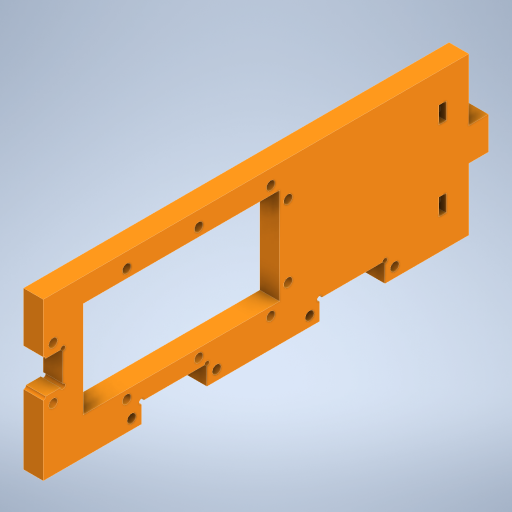
# Autodesk Inventor part: frame_upper2
Saved by Autodesk Inventor 2024 (Build 280153000, 153)
## iProperties
Created: 2024-09-07
Part Number: frame_upper2
Material: PMMA 플라스틱
Document SubType Name: Modeling
Designer: jmha0
Density: 1.188 g/cm^3
Appearance: 주황색
Mass: 30.1586 g
Surface Area: 129.801 cm^2
Volume: 25.386 cm^3
Author: jmha0
Autodesk Inventor part; units mm, degrees
ref_plane "YZ Plane" through (0, 0, 0) normal (1, 0, 0) x (0, 1, 0)
ref_plane "XZ Plane" through (0, 0, 0) normal (0, 1, 0) x (-1, 0, 0)
ref_plane "XY Plane" through (0, 0, 0) normal (0, 0, 1) x (1, 0, 0)
sketch "스케치1" plane through (0, 0, 0) normal (1, 0, 0) x (0, 1, 0)
  line L0 (5.1918, 130.7121) -> (5.1918, 0.7121)
  line L1 (5.1918, 0.7121) -> (11.1918, 0.7121)
  line L2 (11.1918, 130.7121) -> (11.1918, 0.7121)
  line L3 (5.1918, 130.7121) -> (11.1918, 130.7121)
  arc A0 (51.3918, 105.7888) -> (50.8725, 107.4757) centre (48.3918, 105.7888) ccw
  line L4 (50.8725, 107.4757) -> (46.887, 113.3367)
  line L5 (15.6965, 113.3367) -> (11.711, 107.4757)
  arc A1 (11.711, 107.4757) -> (11.1918, 105.7888) centre (14.1918, 105.7888) ccw
  line L6 (11.1918, 105.7888) -> (11.1918, 61.5355)
  arc A2 (11.1918, 61.5355) -> (11.711, 59.8486) centre (14.1918, 61.5355) ccw
  line L7 (11.711, 59.8486) -> (15.3989, 54.4252)
  arc A3 (15.3989, 54.4252) -> (17.8797, 53.1121) centre (17.8797, 56.1121) ccw
  line L8 (17.8797, 53.1121) -> (44.7039, 53.1121)
  arc A4 (44.7039, 53.1121) -> (47.1846, 54.4252) centre (44.7039, 56.1121) ccw
  line L9 (47.1846, 54.4252) -> (50.8725, 59.8486)
  arc A5 (50.8725, 59.8486) -> (51.3918, 61.5355) centre (48.3918, 61.5355) ccw
  line L10 (51.3918, 61.5355) -> (51.3918, 105.7888)
  circle A6 centre (48.5918, 105.2121) radius 1.45
  circle A7 centre (48.5918, 83.2121) radius 1.45
  circle A8 centre (48.5918, 61.2121) radius 1.45
  circle A9 centre (42.2918, 55.9121) radius 1.45
  circle A10 centre (20.2918, 55.9121) radius 1.45
  circle A11 centre (13.9918, 61.2121) radius 1.45
  circle A12 centre (13.9918, 83.2121) radius 1.45
  circle A13 centre (13.9918, 105.2121) radius 1.45
  line L11 (16.5918, 112.7121) -> (16.5918, 59.7121)
  arc A14 (16.5918, 59.7121) -> (17.7918, 58.5121) centre (17.7918, 59.7121) ccw
  line L12 (17.7918, 58.5121) -> (44.7918, 58.5121)
  arc A15 (44.7918, 58.5121) -> (45.9918, 59.7121) centre (44.7918, 59.7121) ccw
  line L13 (45.9918, 59.7121) -> (45.9918, 112.7121)
  line L14 (11.1918, 130.7121) -> (53.1918, 130.7121)
  line L15 (53.1918, 130.7121) -> (53.1918, 0.7121)
  line L16 (53.1918, 0.7121) -> (11.1918, 0.7121)
  line L17 (11.1918, 0.7121) -> (11.1918, 130.7121)
  line L18 (45.9918, 58.5121) -> (16.5918, 58.5121)
  line L19 (16.5918, 58.5121) -> (16.5918, 118.5121)
  line L20 (16.5918, 118.5121) -> (45.9918, 118.5121)
  line L21 (45.9918, 118.5121) -> (45.9918, 58.5121)
  circle A16 centre (48.5918, 105.2121) radius 1.35
  circle A17 centre (48.5918, 83.2121) radius 1.35
  circle A18 centre (48.5918, 61.2121) radius 1.35
  circle A19 centre (42.2918, 55.9121) radius 1.35
  circle A20 centre (20.2918, 55.9121) radius 1.35
  circle A21 centre (13.9918, 61.2121) radius 1.35
  circle A22 centre (13.9918, 83.2121) radius 1.35
  circle A23 centre (13.9918, 105.2121) radius 1.35
  point P0 (31.2918, 101.2121)
  point P1 (32.1918, 130.7121)
  point P2 (45.9918, 59.7121)
  point P3 (17.7918, 58.5121)
  dimension "d9" = 42
  dimension "d10" = 130
  dimension "d11" = 60
  dimension "d12" = 12.2
  dimension "d62" = 0.1
  dimension "d63" = 0.1
  dimension "d64" = 0.1
  dimension "d65" = 0.1
  dimension "d66" = 0.1
  dimension "d67" = 0.1
  dimension "d68" = 0.1
  dimension "d69" = 0.1
  constraints: 44 end point, 24 centre point, 16 point on circle, 4 parallel, 2 perpendicular, 2 point on line, 1 horizontal, 1 midpoint
  measures "d9" distance of L15.end L16.end
  measures "d10" distance of L14.end L15.end
  measures "d11" distance of L18.end L19.end
  measures "d12" distance from line of point (32.192, 130.712) L20
  measures "d62" radial gap between concentric circles of A6 A16
  measures "d63" radial gap between concentric circles of A7 A17
  measures "d64" radial gap between concentric circles of A8 A18
  measures "d65" radial gap between concentric circles of A9 A19
  measures "d66" radial gap between concentric circles of A10 A20
  measures "d67" radial gap between concentric circles of A11 A21
  measures "d68" radial gap between concentric circles of A12 A22
  measures "d69" radial gap between concentric circles of A13 A23
extrude "돌출1" add sketch "스케치1" along normal blind 6 contours L3 L2 L1 L0 | L14 L15 L16 L2 | A6 | A7 | A8 | A9 | A10 | A11 | A12 | A13
sketch "스케치3" plane through (6, 0, 0) normal (1, 0, 0) x (0, 0, -1)
  line L0 (-58.5121, 16.5918) -> (-118.5121, 16.5918) projected
  line L1 (-58.5121, 16.5918) -> (-46.3121, 16.5918)
  line L2 (-130.7121, 5.1918) -> (-0.7121, 5.1918) projected
  line L3 (-46.3121, 5.1918) -> (-26.3121, 5.1918)
  line L4 (-26.3121, 5.1918) -> (-26.3121, 11.1918)
  line L5 (-26.3121, 11.1918) -> (-46.3121, 11.1918)
  line L6 (-46.3121, 11.1918) -> (-46.3121, 5.1918)
  line L7 (-130.7121, 53.1918) -> (-130.7121, 5.1918) projected
  line L8 (-130.7121, 53.1918) -> (-130.7121, 32.1918)
  line L9 (-130.7121, 32.1918) -> (-124.7121, 32.1918)
  line L10 (-124.7121, 32.1918) -> (-124.7121, 42.1918)
  line L11 (-124.7121, 42.1918) -> (-130.7121, 42.1918)
  line L12 (-130.7121, 42.1918) -> (-130.7121, 32.1918)
  line L13 (-124.7121, 32.1918) -> (-130.7121, 32.1918)
  line L14 (-130.7121, 32.1918) -> (-130.7121, 22.1918)
  line L15 (-130.7121, 22.1918) -> (-124.7121, 22.1918)
  line L16 (-124.7121, 22.1918) -> (-124.7121, 32.1918)
  point P0 (0, 0)
  point P1 (-46.3121, 8.1918)
  dimension "d20" = 12.2
  dimension "d21" = 20
  dimension "d22" = 6
  dimension "d25" = 84.4
  dimension "d26" = 48
  dimension "d27" = 21
  dimension "d28" = 6
  dimension "d29" = 10
  dimension "d30" = 10
  constraints: 28 end point, 6 parallel, 4 horizontal, 3 perpendicular, 3 point on line, 1 midpoint
  measures "d20" distance of L0.start L1.end
  measures "d21" distance of L5.end L4.end
  measures "d22" distance of L4.end L3.end
  measures "d25" distance from line of point (-46.312, 8.192) L7
  measures "d26" distance of L7.start L2.start
  measures "d27" distance of L7.start L8.end
  measures "d28" distance of L11.end L10.end
  measures "d29" distance of L10.end L9.end
  measures "d30" distance of L14.end L13.end
extrude "돌출3" cut sketch "스케치3" against normal blind 6 contours L6 L5 L4 L2
sketch "스케치4" plane through (6, 0, 0) normal (1, 0, 0) x (0, 0, -1)
  line L0 (-118.5121, 16.5918) -> (-118.5121, 45.9918) projected
  line L1 (-118.5121, 16.5918) -> (-118.5121, 45.9918) projected
  line L2 (-118.5121, 16.5918) -> (-118.5121, 45.9918) projected
  line L3 (-118.5121, 16.5918) -> (-118.5121, 45.9918) projected
  line L4 (-0.7121, 53.1918) -> (-130.7121, 53.1918) projected
  line L5 (-130.7121, 53.1918) -> (-130.7121, 36.1918)
  line L6 (-130.7121, 53.1918) -> (-130.7121, 5.1918) projected
  line L7 (-130.7121, 26.1918) -> (-130.7121, 36.1918)
  line L8 (-0.7121, 53.1918) -> (-130.7121, 53.1918) projected
  line L9 (-46.3121, 11.1918) -> (-26.3121, 11.1918) projected
  line L10 (-118.5121, 16.5918) -> (-118.5121, 45.9918) projected
  line L11 (-118.5121, 45.9918) -> (-58.5121, 45.9918) projected
  line L12 (-58.5121, 45.9918) -> (-58.5121, 16.5918) projected
  line L13 (-58.5121, 16.5918) -> (-118.5121, 16.5918) projected
  line L14 (-139.9357, 113.6265) -> (-199.9357, 113.6265)
  line L15 (-139.9357, 113.6265) -> (-127.7357, 113.6265)
  line L16 (-212.1357, 102.2265) -> (-82.1357, 102.2265)
  line L17 (-127.7357, 102.2265) -> (-107.7357, 102.2265)
  line L18 (-107.7357, 102.2265) -> (-107.7357, 108.2265)
  line L19 (-107.7357, 108.2265) -> (-127.7357, 108.2265)
  line L20 (-127.7357, 108.2265) -> (-127.7357, 102.2265)
  line L21 (-212.1357, 150.2265) -> (-212.1357, 102.2265)
  line L22 (-212.1357, 150.2265) -> (-212.1357, 129.2265)
  line L23 (-212.1357, 129.2265) -> (-206.1357, 129.2265)
  line L24 (-206.1357, 129.2265) -> (-206.1357, 139.2265)
  line L25 (-206.1357, 139.2265) -> (-212.1357, 139.2265)
  line L26 (-212.1357, 139.2265) -> (-212.1357, 129.2265)
  line L27 (-206.1357, 129.2265) -> (-212.1357, 129.2265)
  line L28 (-212.1357, 129.2265) -> (-212.1357, 119.2265)
  line L29 (-212.1357, 119.2265) -> (-206.1357, 119.2265)
  line L30 (-206.1357, 119.2265) -> (-206.1357, 129.2265)
  line L31 (-130.7121, 53.1918) -> (-130.7121, 37.1918)
  line L32 (-130.7121, 37.1918) -> (-124.7121, 37.1918)
  line L33 (-124.7121, 37.1918) -> (-124.7121, 27.1918)
  line L34 (-124.7121, 27.1918) -> (-130.7121, 27.1918)
  line L35 (-130.7121, 27.1918) -> (-130.7121, 37.1918)
  line L36 (-26.3121, 11.1918) -> (-26.3121, 5.1918) projected
  line L37 (-26.3121, 5.1918) -> (-0.7121, 5.1918) projected
  line L38 (-0.7121, 5.1918) -> (-0.7121, 53.1918) projected
  line L39 (-130.7121, 53.1918) -> (-130.7121, 5.1918) projected
  line L40 (-130.7121, 5.1918) -> (-46.3121, 5.1918) projected
  line L41 (-46.3121, 5.1918) -> (-46.3121, 11.1918) projected
  point P0 (0, 0)
  point P1 (-81.4235, 97.0347)
  point P2 (-127.7357, 105.2265)
  dimension "d34" = 12.2
  dimension "d35" = 20
  dimension "d36" = 6
  dimension "d37" = 84.4
  dimension "d38" = 48
  dimension "d39" = 21
  dimension "d40" = 6
  dimension "d41" = 10
  dimension "d42" = 10
  dimension "d43" = 16
  dimension "d44" = 6
  dimension "d45" = 10
  constraints: 48 end point, 8 parallel, 5 horizontal, 4 perpendicular, 4 point on line, 1 midpoint
  measures "d34" distance of L14.start L15.end
  measures "d35" distance of L19.end L18.end
  measures "d36" distance of L18.end L17.end
  measures "d37" distance from line of point (-127.736, 105.226) L21
  measures "d38" distance of L21.start L16.start
  measures "d39" distance of L21.start L22.end
  measures "d40" distance of L25.end L24.end
  measures "d41" distance of L24.end L23.end
  measures "d42" distance of L28.end L27.end
  measures "d43" distance of L8.end L31.end
  measures "d44" distance of L33.end L34.end
  measures "d45" distance of L32.end L33.end
extrude "돌출4" cut sketch "스케치4" against normal blind 6 contours L32 L33 L34 L6 L5
sketch "스케치6" plane through (6, 0, 0) normal (1, 0, 0) x (0, 0, -1)
  line L0 (-118.5121, 16.5918) -> (-118.5121, 45.9918) projected
  line L1 (-118.5121, 45.9918) -> (-58.5121, 45.9918) projected
  line L2 (-58.5121, 45.9918) -> (-58.5121, 16.5918) projected
  line L3 (-58.5121, 16.5918) -> (-118.5121, 16.5918) projected
  line L4 (-130.7121, 37.1918) -> (-124.7121, 37.1918) projected
  line L5 (-124.7121, 37.1918) -> (-124.7121, 27.1918) projected
  line L6 (-124.7121, 27.1918) -> (-130.7121, 27.1918) projected
  line L7 (-46.3121, 11.1918) -> (-26.3121, 11.1918) projected
  line L8 (-0.7121, 53.1918) -> (-130.7121, 53.1918) projected
  line L9 (-130.7121, 53.1918) -> (-130.7121, 37.1918) projected
  line L10 (-130.7121, 37.1918) -> (-124.7121, 37.1918)
  line L11 (-124.7121, 37.1918) -> (-124.7121, 43.1918)
  line L12 (-124.7121, 43.1918) -> (-130.7121, 43.1918)
  line L13 (-130.7121, 43.1918) -> (-130.7121, 37.1918)
  line L14 (-130.7121, 27.1918) -> (-124.7121, 27.1918)
  line L15 (-124.7121, 27.1918) -> (-124.7121, 21.1918)
  line L16 (-124.7121, 21.1918) -> (-130.7121, 21.1918)
  line L17 (-130.7121, 21.1918) -> (-130.7121, 27.1918)
  circle A0 centre (-127.7121, 40.1918) radius 1.35
  circle A1 centre (-127.7121, 24.1918) radius 1.35
  line L18 (-130.7121, 27.1918) -> (-130.7121, 5.1918) projected
  line L19 (-130.7121, 5.1918) -> (-46.3121, 5.1918) projected
  line L20 (-46.3121, 5.1918) -> (-46.3121, 11.1918) projected
  line L21 (-26.3121, 11.1918) -> (-26.3121, 5.1918) projected
  line L22 (-26.3121, 5.1918) -> (-0.7121, 5.1918) projected
  line L23 (-0.7121, 5.1918) -> (-0.7121, 53.1918) projected
  point P0 (0, 0)
  dimension "d48" = 6
  dimension "d49" = 6
  dimension "d50" = 2.7
  dimension "d51" = 2.7
  constraints: 16 end point, 4 parallel, 2 centre point, 2 horizontal, 2 perpendicular, 1 point on line
  measures "d48" distance of L11.end L10.end
  measures "d49" distance of L14.end L15.end
  measures "d50" diameter of A0
  measures "d51" diameter of A1
extrude "돌출5" cut sketch "스케치6" against normal blind 6 contours A0 | A1
sketch "스케치7" plane through (6, 0, 0) normal (1, 0, 0) x (0, 0, -1)
  circle A0 centre (-127.7121, 24.1918) radius 1.35 projected
  circle A1 centre (-127.7121, 40.1918) radius 1.35 projected
  line L0 (-118.5121, 16.5918) -> (-118.5121, 45.9918) projected
  line L1 (-118.5121, 45.9918) -> (-58.5121, 45.9918) projected
  line L2 (-58.5121, 45.9918) -> (-58.5121, 16.5918) projected
  line L3 (-58.5121, 16.5918) -> (-118.5121, 16.5918) projected
  line L4 (-130.7121, 37.1918) -> (-124.7121, 37.1918) projected
  line L5 (-124.7121, 37.1918) -> (-124.7121, 27.1918) projected
  line L6 (-124.7121, 27.1918) -> (-130.7121, 27.1918) projected
  line L7 (-46.3121, 11.1918) -> (-26.3121, 11.1918) projected
  line L8 (-0.7121, 53.1918) -> (-130.7121, 53.1918) projected
  line L9 (-130.7121, 53.1918) -> (-130.7121, 37.1918) projected
  line L10 (-26.3121, 5.1918) -> (-20.3121, 5.1918)
  line L11 (-20.3121, 5.1918) -> (-20.3121, 11.1918)
  line L12 (-20.3121, 11.1918) -> (-26.3121, 11.1918)
  line L13 (-26.3121, 11.1918) -> (-26.3121, 5.1918)
  line L14 (-46.3121, 5.1918) -> (-52.3121, 5.1918)
  line L15 (-52.3121, 5.1918) -> (-52.3121, 11.1918)
  line L16 (-52.3121, 11.1918) -> (-46.3121, 11.1918)
  line L17 (-46.3121, 11.1918) -> (-46.3121, 5.1918)
  circle A2 centre (-49.3121, 8.1918) radius 1.35
  circle A3 centre (-23.3121, 8.1918) radius 1.35
  line L18 (-130.7121, 27.1918) -> (-130.7121, 5.1918) projected
  line L19 (-130.7121, 5.1918) -> (-46.3121, 5.1918) projected
  line L20 (-46.3121, 5.1918) -> (-46.3121, 11.1918) projected
  line L21 (-26.3121, 11.1918) -> (-26.3121, 5.1918) projected
  line L22 (-26.3121, 5.1918) -> (-0.7121, 5.1918) projected
  line L23 (-0.7121, 5.1918) -> (-0.7121, 53.1918) projected
  point P0 (0, 0)
  dimension "d54" = 6
  dimension "d55" = 6
  dimension "d56" = 6
  dimension "d57" = 6
  dimension "d58" = 2.7
  dimension "d59" = 2.7
  constraints: 16 end point, 4 parallel, 2 centre point, 2 horizontal, 2 perpendicular
  measures "d54" distance of L12.end L11.end
  measures "d55" distance of L11.end L10.end
  measures "d56" distance of L15.end L16.end
  measures "d57" distance of L14.end L15.end
  measures "d58" diameter of A2
  measures "d59" diameter of A3
extrude "돌출6" cut sketch "스케치7" against normal blind 6 contours A2 | A3
sketch "스케치8" plane through (0, 5.1918, 0.7121) normal (0, 0, -1) x (-1, 0, 0)
  line L0 (0, 0) -> (0, 48) projected
  line L1 (0, 48) -> (-6, 48) projected
  line L2 (-6, 0) -> (-6, 48) projected
  line L3 (0, 0) -> (-6, 0) projected
  line L4 (-6, 0) -> (-6, 48) projected
  line L5 (-6, 48) -> (-6, 36)
  line L6 (-6, 36) -> (-6, 12)
  circle A0 centre (-3, 36) radius 1.35
  circle A1 centre (-3, 12) radius 1.35
  point P0 (0, -5.1918)
  dimension "d70" = 48
  dimension "d71" = 6
  dimension "d72" = 12
  dimension "d73" = 24
  dimension "d74" = 2.7
  dimension "d75" = 2.7
  constraints: 4 end point, 2 centre point, 2 point on line
  measures "d70" distance of L2.start L1.end
  measures "d71" distance of L0.end L1.end
  measures "d72" distance of L1.end L5.end
  measures "d73" distance of L5.end L6.end
  measures "d74" diameter of A0
  measures "d75" diameter of A1
extrude "돌출7" cut sketch "스케치8" against normal blind 16 contours A0 | A1
sketch "스케치10" plane through (6, 0, 0) normal (1, 0, 0) x (0, 0, -1)
  line L0 (-16.7121, 42.5418) -> (-16.7121, 39.8418) projected
  line L1 (-16.7121, 18.5418) -> (-16.7121, 15.8418) projected
  line L2 (-0.7121, 18.5418) -> (-0.7121, 15.8418) projected
  line L3 (-0.7121, 42.5418) -> (-0.7121, 39.8418) projected
  line L4 (-16.7121, 42.5418) -> (-16.7121, 39.8418) projected
  line L5 (-16.7121, 18.5418) -> (-16.7121, 15.8418) projected
  line L6 (-16.7121, 42.5418) -> (-16.7121, 39.8418) projected
  line L7 (-0.7121, 42.5418) -> (-0.7121, 39.8418) projected
  line L8 (-16.7121, 18.5418) -> (-16.7121, 15.8418) projected
  line L9 (-0.7121, 18.5418) -> (-0.7121, 15.8418) projected
  line L10 (-0.7121, 42.5418) -> (-16.7121, 42.5418) projected
  line L11 (-0.7121, 39.8418) -> (-16.7121, 39.8418) projected
  line L12 (-0.7121, 18.5418) -> (-16.7121, 18.5418) projected
  circle A0 centre (-23.3121, 8.1918) radius 1.35 projected
  circle A1 centre (-49.3121, 8.1918) radius 1.35 projected
  circle A2 centre (-127.7121, 24.1918) radius 1.35 projected
  circle A3 centre (-127.7121, 40.1918) radius 1.35 projected
  line L13 (-118.5121, 16.5918) -> (-118.5121, 45.9918) projected
  line L14 (-118.5121, 45.9918) -> (-58.5121, 45.9918) projected
  line L15 (-58.5121, 45.9918) -> (-58.5121, 16.5918) projected
  line L16 (-58.5121, 16.5918) -> (-118.5121, 16.5918) projected
  circle A4 centre (-105.2121, 13.9918) radius 1.35 projected
  circle A5 centre (-83.2121, 13.9918) radius 1.35 projected
  circle A6 centre (-61.2121, 13.9918) radius 1.35 projected
  circle A7 centre (-55.9121, 20.2918) radius 1.35 projected
  circle A8 centre (-55.9121, 42.2918) radius 1.35 projected
  circle A9 centre (-61.2121, 48.5918) radius 1.35 projected
  circle A10 centre (-83.2121, 48.5918) radius 1.35 projected
  circle A11 centre (-105.2121, 48.5918) radius 1.35 projected
  line L17 (-130.7121, 37.1918) -> (-124.7121, 37.1918) projected
  line L18 (-124.7121, 37.1918) -> (-124.7121, 27.1918) projected
  line L19 (-124.7121, 27.1918) -> (-130.7121, 27.1918) projected
  line L20 (-130.7121, 27.1918) -> (-130.7121, 5.1918) projected
  line L21 (-130.7121, 5.1918) -> (-46.3121, 5.1918) projected
  line L22 (-46.3121, 5.1918) -> (-46.3121, 11.1918) projected
  line L23 (-46.3121, 11.1918) -> (-26.3121, 11.1918) projected
  line L24 (-26.3121, 11.1918) -> (-26.3121, 5.1918) projected
  line L25 (-26.3121, 5.1918) -> (-0.7121, 5.1918) projected
  line L26 (-0.7121, 5.1918) -> (-0.7121, 53.1918) projected
  line L27 (-0.7121, 53.1918) -> (-130.7121, 53.1918) projected
  line L28 (-130.7121, 53.1918) -> (-130.7121, 37.1918) projected
  line L29 (-0.7121, 15.8418) -> (-16.7121, 15.8418) projected
  line L30 (-9.8121, 38.9418) -> (-7.6121, 38.9418)
  line L31 (-7.6121, 38.9418) -> (-7.6121, 44.1418)
  line L32 (-7.6121, 44.1418) -> (-9.8121, 44.1418)
  line L33 (-9.8121, 44.1418) -> (-9.8121, 38.9418)
  line L34 (-9.8121, 38.9418) -> (-7.6121, 44.1418) construction
  line L35 (-7.6121, 38.9418) -> (-9.8121, 44.1418) construction
  line L36 (-9.8121, 14.5918) -> (-7.6121, 14.5918)
  line L37 (-7.6121, 14.5918) -> (-7.6121, 19.7918)
  line L38 (-7.6121, 19.7918) -> (-9.8121, 19.7918)
  line L39 (-9.8121, 19.7918) -> (-9.8121, 14.5918)
  line L40 (-9.8121, 14.5918) -> (-7.6121, 19.7918) construction
  line L41 (-7.6121, 14.5918) -> (-9.8121, 19.7918) construction
  point P0 (0, 0)
  point P1 (-8.7121, 41.5418)
  point P2 (-8.7121, 17.1918)
  dimension "d83" = 2.2
  dimension "d84" = 5.2
  dimension "d85" = 2.2
  dimension "d86" = 5.2
  constraints: 24 end point, 4 midpoint, 4 parallel, 2 horizontal, 2 perpendicular
  measures "d83" distance of L32.end L31.end
  measures "d84" distance of L31.end L30.end
  measures "d85" distance of L38.end L37.end
  measures "d86" distance of L37.end L36.end
extrude "돌출9" cut sketch "스케치10" against normal blind 16 contours L33 L32 L31 L10 | L10 L31 L11 L33 | L11 L31 L30 L33 | L37 L29 L39 L12 | L12 L39 L38 L37 | L37 L36 L39 L29
sketch "스케치11" plane through (0, 5.1918, 0.7121) normal (0, 0, -1) x (-1, 0, 0)
  circle A0 centre (-3, 12) radius 1.35 projected
  circle A1 centre (-3, 36) radius 1.35 projected
  line L0 (0, 0) -> (0, 48) projected
  line L1 (0, 48) -> (-6, 48) projected
  line L2 (-6, 0) -> (-6, 48) projected
  line L3 (0, 0) -> (-6, 0) projected
  line L4 (-6, 19) -> (0, 19)
  line L5 (0, 19) -> (0, 29)
  line L6 (0, 29) -> (-6, 29)
  line L7 (-6, 29) -> (-6, 19)
  line L8 (-6, 19) -> (0, 29) construction
  line L9 (0, 19) -> (-6, 29) construction
  point P0 (0, -5.1918)
  point P1 (-3, 24)
  dimension "d89" = 10
  constraints: 12 end point, 2 midpoint, 2 parallel, 1 horizontal, 1 perpendicular, 1 point on line
  measures "d89" distance of L5.end L4.end
extrude "돌출10" add sketch "스케치11" along normal blind 6 contours L4 L2 L6 L0
sketch "스케치12" plane through (6, 0, 0) normal (1, 0, 0) x (0, 0, -1)
  line L0 (-7.6121, 14.5918) -> (-9.8121, 14.5918) projected
  line L1 (-9.8121, 14.5918) -> (-9.8121, 19.7918) projected
  line L2 (-9.8121, 19.7918) -> (-7.6121, 19.7918) projected
  line L3 (-7.6121, 19.7918) -> (-7.6121, 14.5918) projected
  line L4 (-7.6121, 38.9418) -> (-9.8121, 38.9418) projected
  line L5 (-9.8121, 38.9418) -> (-9.8121, 44.1418) projected
  line L6 (-9.8121, 44.1418) -> (-7.6121, 44.1418) projected
  line L7 (-7.6121, 44.1418) -> (-7.6121, 38.9418) projected
  circle A0 centre (-23.3121, 8.1918) radius 1.35 projected
  circle A1 centre (-49.3121, 8.1918) radius 1.35 projected
  circle A2 centre (-127.7121, 24.1918) radius 1.35 projected
  circle A3 centre (-127.7121, 40.1918) radius 1.35 projected
  line L8 (-118.5121, 16.5918) -> (-118.5121, 45.9918) projected
  line L9 (-118.5121, 45.9918) -> (-58.5121, 45.9918) projected
  line L10 (-58.5121, 45.9918) -> (-58.5121, 16.5918) projected
  line L11 (-58.5121, 16.5918) -> (-118.5121, 16.5918) projected
  circle A4 centre (-105.2121, 13.9918) radius 1.35 projected
  circle A5 centre (-83.2121, 13.9918) radius 1.35 projected
  circle A6 centre (-61.2121, 13.9918) radius 1.35 projected
  circle A7 centre (-55.9121, 20.2918) radius 1.35 projected
  circle A8 centre (-55.9121, 42.2918) radius 1.35 projected
  circle A9 centre (-61.2121, 48.5918) radius 1.35 projected
  circle A10 centre (-83.2121, 48.5918) radius 1.35 projected
  circle A11 centre (-105.2121, 48.5918) radius 1.35 projected
  line L12 (-130.7121, 37.1918) -> (-124.7121, 37.1918) projected
  line L13 (-124.7121, 37.1918) -> (-124.7121, 27.1918) projected
  line L14 (-124.7121, 27.1918) -> (-130.7121, 27.1918) projected
  line L15 (-130.7121, 27.1918) -> (-130.7121, 5.1918) projected
  line L16 (-130.7121, 5.1918) -> (-46.3121, 5.1918) projected
  line L17 (-46.3121, 5.1918) -> (-46.3121, 11.1918) projected
  line L18 (-46.3121, 11.1918) -> (-26.3121, 11.1918) projected
  line L19 (-26.3121, 11.1918) -> (-26.3121, 5.1918) projected
  line L20 (-26.3121, 5.1918) -> (-0.7121, 5.1918) projected
  line L21 (-0.7121, 5.1918) -> (-0.7121, 24.1918) projected
  line L22 (-0.7121, 24.1918) -> (5.2879, 24.1918) projected
  line L23 (5.2879, 34.1918) -> (5.2879, 24.1918) projected
  line L24 (-0.7121, 34.1918) -> (5.2879, 34.1918) projected
  line L25 (-0.7121, 34.1918) -> (-0.7121, 53.1918) projected
  line L26 (-0.7121, 53.1918) -> (-130.7121, 53.1918) projected
  line L27 (-130.7121, 53.1918) -> (-130.7121, 37.1918) projected
  circle A12 centre (-46.3121, 11.1918) radius 0.75
  circle A13 centre (-26.3121, 11.1918) radius 0.75
  circle A14 centre (-26.3121, 5.1918) radius 0.75
  line L28 (-130.7121, 5.1918) -> (-46.3121, 5.1918) projected
  circle A15 centre (-46.3121, 5.1918) radius 0.75
  circle A16 centre (-124.7121, 37.1918) radius 0.75
  circle A17 centre (-130.7121, 37.1918) radius 0.75
  line L29 (-130.7121, 27.1918) -> (-130.7121, 5.1918) projected
  circle A18 centre (-130.7121, 27.1918) radius 0.75
  circle A19 centre (-124.7121, 27.1918) radius 0.75
  point P0 (0, 0)
  point P1 (-124.7121, 27.9418)
  point P2 (-125.4621, 27.1918)
  point P3 (-129.9621, 37.1918)
  point P4 (-130.7121, 37.9418)
  point P5 (-124.7121, 36.4418)
  point P6 (-125.4621, 37.1918)
  point P7 (-45.5621, 11.1918)
  point P8 (-46.3121, 10.4418)
  point P9 (-26.3121, 10.4418)
  point P10 (-27.0621, 11.1918)
  dimension "d92" = 1.5
  dimension "d93" = 1.5
  dimension "d94" = 1.5
  dimension "d95" = 1.5
  dimension "d96" = 1.5
  dimension "d97" = 1.5
  dimension "d98" = 1.5
  dimension "d99" = 1.5
  constraints: 8 centre point, 8 coincident
  measures "d92" diameter of A12
  measures "d93" diameter of A13
  measures "d94" diameter of A14
  measures "d95" diameter of A15
  measures "d96" diameter of A16
  measures "d97" diameter of A17
  measures "d98" diameter of A18
  measures "d99" diameter of A19
extrude "돌출11" cut sketch "스케치12" against normal blind 6 contours L27 A17 L12 | A16 L13 L12 | A19 L14 L13 | A18 L15 L14 | L14 L15 A18 | A15 L17 L16 | L16 L17 A15 | A14 L19 L20 | L20 L19 A14 | A12 L18 L17 | L19 L18 A13 picked at (-130.4478, 37.6125) picked at (-124.9428, 37.6313) picked at (-124.9428, 26.7523) picked at (-46.3735, 10.6994) picked at (-26.8048, 11.2516)
sketch "스케치13" plane through (6, 0, 0) normal (1, 0, 0) x (0, 0, -1)
  circle A0 centre (-105.2121, 48.5918) radius 1.35 projected
  circle A1 centre (-83.2121, 48.5918) radius 1.35 projected
  circle A2 centre (-61.2121, 48.5918) radius 1.35 projected
  circle A3 centre (-55.9121, 42.2918) radius 1.35 projected
  circle A4 centre (-55.9121, 20.2918) radius 1.35 projected
  circle A5 centre (-61.2121, 13.9918) radius 1.35 projected
  circle A6 centre (-83.2121, 13.9918) radius 1.35 projected
  circle A7 centre (-105.2121, 13.9918) radius 1.35 projected
  line L0 (-118.5121, 16.5918) -> (-118.5121, 45.9918) projected
  line L1 (-118.5121, 45.9918) -> (-58.5121, 45.9918) projected
  line L2 (-58.5121, 45.9918) -> (-58.5121, 16.5918) projected
  line L3 (-58.5121, 16.5918) -> (-118.5121, 16.5918) projected
  circle A8 centre (-127.7121, 40.1918) radius 1.35 projected
  circle A9 centre (-127.7121, 24.1918) radius 1.35 projected
  circle A10 centre (-49.3121, 8.1918) radius 1.35 projected
  circle A11 centre (-23.3121, 8.1918) radius 1.35 projected
  line L4 (-7.6121, 38.9418) -> (-9.8121, 38.9418) projected
  line L5 (-9.8121, 38.9418) -> (-9.8121, 44.1418) projected
  line L6 (-9.8121, 44.1418) -> (-7.6121, 44.1418) projected
  line L7 (-7.6121, 44.1418) -> (-7.6121, 38.9418) projected
  line L8 (-7.6121, 14.5918) -> (-9.8121, 14.5918) projected
  line L9 (-9.8121, 14.5918) -> (-9.8121, 19.7918) projected
  line L10 (-9.8121, 19.7918) -> (-7.6121, 19.7918) projected
  line L11 (-7.6121, 19.7918) -> (-7.6121, 14.5918) projected
  arc A12 (-45.5621, 11.1918) -> (-46.3121, 10.4418) centre (-46.3121, 11.1918) ccw projected
  line L12 (-45.5621, 11.1918) -> (-27.0621, 11.1918) projected
  arc A13 (-26.3121, 10.4418) -> (-27.0621, 11.1918) centre (-26.3121, 11.1918) ccw projected
  line L13 (-26.3121, 10.4418) -> (-26.3121, 5.9418) projected
  arc A14 (-25.5621, 5.1918) -> (-26.3121, 5.9418) centre (-26.3121, 5.1918) ccw projected
  line L14 (-25.5621, 5.1918) -> (-0.7121, 5.1918) projected
  line L15 (-0.7121, 5.1918) -> (-0.7121, 24.1918) projected
  line L16 (-0.7121, 24.1918) -> (5.2879, 24.1918) projected
  line L17 (5.2879, 34.1918) -> (5.2879, 24.1918) projected
  line L18 (-0.7121, 34.1918) -> (5.2879, 34.1918) projected
  line L19 (-0.7121, 34.1918) -> (-0.7121, 53.1918) projected
  line L20 (-0.7121, 53.1918) -> (-130.7121, 53.1918) projected
  line L21 (-130.7121, 53.1918) -> (-130.7121, 37.9418) projected
  arc A15 (-129.9621, 37.1918) -> (-130.7121, 37.9418) centre (-130.7121, 37.1918) ccw projected
  line L22 (-129.9621, 37.1918) -> (-125.4621, 37.1918) projected
  arc A16 (-124.7121, 36.4418) -> (-125.4621, 37.1918) centre (-124.7121, 37.1918) ccw projected
  line L23 (-124.7121, 36.4418) -> (-124.7121, 27.9418) projected
  arc A17 (-125.4621, 27.1918) -> (-124.7121, 27.9418) centre (-124.7121, 27.1918) ccw projected
  line L24 (-125.4621, 27.1918) -> (-129.9621, 27.1918) projected
  arc A18 (-130.7121, 26.4418) -> (-129.9621, 27.1918) centre (-130.7121, 27.1918) ccw projected
  line L25 (-130.7121, 26.4418) -> (-130.7121, 5.1918) projected
  line L26 (-130.7121, 5.1918) -> (-47.0621, 5.1918) projected
  arc A19 (-46.3121, 5.9418) -> (-47.0621, 5.1918) centre (-46.3121, 5.1918) ccw projected
  line L27 (-46.3121, 5.9418) -> (-46.3121, 10.4418) projected
  line L28 (-130.7121, 5.1918) -> (-100.7121, 5.1918)
  line L29 (-100.7121, 5.1918) -> (-80.7121, 5.1918)
  line L30 (-80.7121, 5.1918) -> (-80.7121, 11.1918)
  line L31 (-80.7121, 11.1918) -> (-100.7121, 11.1918)
  line L32 (-100.7121, 11.1918) -> (-100.7121, 5.1918)
  line L33 (-100.7121, 8.1918) -> (-103.7121, 8.1918)
  line L34 (-103.7121, 8.1918) -> (-77.7121, 8.1918)
  circle A20 centre (-103.7121, 8.1918) radius 1.35
  circle A21 centre (-77.7121, 8.1918) radius 1.35
  point P0 (0, 0)
  dimension "d102" = 30
  dimension "d103" = 20
  dimension "d104" = 6
  dimension "d105" = 3
  dimension "d106" = 26
  dimension "d107" = 2.7
  dimension "d108" = 2.7
  constraints: 14 end point, 3 parallel, 2 centre point, 2 coincident, 2 point on line, 1 horizontal, 1 midpoint, 1 perpendicular
  measures "d102" distance of L25.end L28.end
  measures "d103" distance of L31.end L30.end
  measures "d104" distance of L30.end L29.end
  measures "d105" distance of L33.start L33.end
  measures "d106" distance of L33.end L34.end
  measures "d107" diameter of A20
  measures "d108" diameter of A21
extrude "돌출12" cut sketch "스케치13" against normal blind 6 contours L26 L32 L34 L30 | L34 L32 L31 L30 | A20 | A21
sketch "스케치14" plane through (6, 0, 0) normal (1, 0, 0) x (0, 0, -1)
  line L0 (-80.7121, 11.1918) -> (-80.7121, 5.1918) projected
  line L1 (-80.7121, 5.1918) -> (-47.0621, 5.1918) projected
  arc A0 (-46.3121, 5.9418) -> (-47.0621, 5.1918) centre (-46.3121, 5.1918) ccw projected
  line L2 (-46.3121, 5.9418) -> (-46.3121, 10.4418) projected
  arc A1 (-45.5621, 11.1918) -> (-46.3121, 10.4418) centre (-46.3121, 11.1918) ccw projected
  line L3 (-45.5621, 11.1918) -> (-27.0621, 11.1918) projected
  arc A2 (-26.3121, 10.4418) -> (-27.0621, 11.1918) centre (-26.3121, 11.1918) ccw projected
  line L4 (-26.3121, 10.4418) -> (-26.3121, 5.9418) projected
  arc A3 (-25.5621, 5.1918) -> (-26.3121, 5.9418) centre (-26.3121, 5.1918) ccw projected
  line L5 (-25.5621, 5.1918) -> (-0.7121, 5.1918) projected
  line L6 (-0.7121, 5.1918) -> (-0.7121, 24.1918) projected
  line L7 (-0.7121, 24.1918) -> (5.2879, 24.1918) projected
  line L8 (5.2879, 34.1918) -> (5.2879, 24.1918) projected
  line L9 (-0.7121, 34.1918) -> (5.2879, 34.1918) projected
  line L10 (-0.7121, 34.1918) -> (-0.7121, 53.1918) projected
  line L11 (-0.7121, 53.1918) -> (-130.7121, 53.1918) projected
  line L12 (-130.7121, 53.1918) -> (-130.7121, 37.9418) projected
  arc A4 (-129.9621, 37.1918) -> (-130.7121, 37.9418) centre (-130.7121, 37.1918) ccw projected
  line L13 (-129.9621, 37.1918) -> (-125.4621, 37.1918) projected
  arc A5 (-124.7121, 36.4418) -> (-125.4621, 37.1918) centre (-124.7121, 37.1918) ccw projected
  line L14 (-124.7121, 36.4418) -> (-124.7121, 27.9418) projected
  arc A6 (-125.4621, 27.1918) -> (-124.7121, 27.9418) centre (-124.7121, 27.1918) ccw projected
  line L15 (-125.4621, 27.1918) -> (-129.9621, 27.1918) projected
  arc A7 (-130.7121, 26.4418) -> (-129.9621, 27.1918) centre (-130.7121, 27.1918) ccw projected
  line L16 (-130.7121, 26.4418) -> (-130.7121, 5.1918) projected
  line L17 (-130.7121, 5.1918) -> (-100.7121, 5.1918) projected
  line L18 (-100.7121, 5.1918) -> (-100.7121, 11.1918) projected
  line L19 (-100.7121, 11.1918) -> (-80.7121, 11.1918) projected
  circle A8 centre (-77.7121, 8.1918) radius 1.35 projected
  circle A9 centre (-103.7121, 8.1918) radius 1.35 projected
  circle A10 centre (-105.2121, 48.5918) radius 1.35 projected
  circle A11 centre (-83.2121, 48.5918) radius 1.35 projected
  circle A12 centre (-61.2121, 48.5918) radius 1.35 projected
  circle A13 centre (-55.9121, 42.2918) radius 1.35 projected
  circle A14 centre (-55.9121, 20.2918) radius 1.35 projected
  circle A15 centre (-61.2121, 13.9918) radius 1.35 projected
  circle A16 centre (-83.2121, 13.9918) radius 1.35 projected
  circle A17 centre (-105.2121, 13.9918) radius 1.35 projected
  line L20 (-118.5121, 16.5918) -> (-118.5121, 45.9918) projected
  line L21 (-118.5121, 45.9918) -> (-58.5121, 45.9918) projected
  line L22 (-58.5121, 45.9918) -> (-58.5121, 16.5918) projected
  line L23 (-58.5121, 16.5918) -> (-118.5121, 16.5918) projected
  circle A18 centre (-127.7121, 40.1918) radius 1.35 projected
  circle A19 centre (-127.7121, 24.1918) radius 1.35 projected
  circle A20 centre (-49.3121, 8.1918) radius 1.35 projected
  circle A21 centre (-23.3121, 8.1918) radius 1.35 projected
  line L24 (-7.6121, 38.9418) -> (-9.8121, 38.9418) projected
  line L25 (-9.8121, 38.9418) -> (-9.8121, 44.1418) projected
  line L26 (-9.8121, 44.1418) -> (-7.6121, 44.1418) projected
  line L27 (-7.6121, 44.1418) -> (-7.6121, 38.9418) projected
  line L28 (-7.6121, 14.5918) -> (-9.8121, 14.5918) projected
  line L29 (-9.8121, 14.5918) -> (-9.8121, 19.7918) projected
  line L30 (-9.8121, 19.7918) -> (-7.6121, 19.7918) projected
  line L31 (-7.6121, 19.7918) -> (-7.6121, 14.5918) projected
  circle A22 centre (-100.7121, 11.1918) radius 0.75
  circle A23 centre (-100.7121, 5.1918) radius 0.75
  line L32 (-100.7121, 11.1918) -> (-80.7121, 11.1918) projected
  circle A24 centre (-80.7121, 11.1918) radius 0.75
  circle A25 centre (-80.7121, 5.1918) radius 0.75
  point P0 (0, 0)
  point P1 (-80.7121, 10.4418)
  point P2 (-81.4621, 11.1918)
  point P3 (-99.9621, 11.1918)
  point P4 (-100.7121, 10.4418)
  dimension "d111" = 1.5
  dimension "d112" = 1.5
  dimension "d113" = 1.5
  dimension "d114" = 1.5
  constraints: 4 centre point, 4 coincident
  measures "d111" diameter of A22
  measures "d112" diameter of A23
  measures "d113" diameter of A24
  measures "d114" diameter of A25
extrude "돌출13" cut sketch "스케치14" against normal blind 6 contours L19 A24 L0 | A25 L1 L0 | L0 L1 A25 | L19 L18 A22 | A23 L17 L18 | L18 L17 A23 picked at (-81.2048, 11.2516) picked at (-100.7326, 11.6875)
sketch "스케치15" plane through (6, 0, 0) normal (1, 0, 0) x (0, 0, -1)
  arc A0 (-80.7121, 10.4418) -> (-81.4621, 11.1918) centre (-80.7121, 11.1918) ccw projected
  line L0 (-80.7121, 10.4418) -> (-80.7121, 5.9418) projected
  arc A1 (-79.9621, 5.1918) -> (-80.7121, 5.9418) centre (-80.7121, 5.1918) ccw projected
  line L1 (-79.9621, 5.1918) -> (-47.0621, 5.1918) projected
  arc A2 (-46.3121, 5.9418) -> (-47.0621, 5.1918) centre (-46.3121, 5.1918) ccw projected
  line L2 (-46.3121, 5.9418) -> (-46.3121, 10.4418) projected
  arc A3 (-45.5621, 11.1918) -> (-46.3121, 10.4418) centre (-46.3121, 11.1918) ccw projected
  line L3 (-45.5621, 11.1918) -> (-27.0621, 11.1918) projected
  arc A4 (-26.3121, 10.4418) -> (-27.0621, 11.1918) centre (-26.3121, 11.1918) ccw projected
  line L4 (-26.3121, 10.4418) -> (-26.3121, 5.9418) projected
  arc A5 (-25.5621, 5.1918) -> (-26.3121, 5.9418) centre (-26.3121, 5.1918) ccw projected
  line L5 (-25.5621, 5.1918) -> (-0.7121, 5.1918) projected
  line L6 (-0.7121, 5.1918) -> (-0.7121, 24.1918) projected
  line L7 (-0.7121, 24.1918) -> (5.2879, 24.1918) projected
  line L8 (5.2879, 34.1918) -> (5.2879, 24.1918) projected
  line L9 (-0.7121, 34.1918) -> (5.2879, 34.1918) projected
  line L10 (-0.7121, 34.1918) -> (-0.7121, 53.1918) projected
  line L11 (-0.7121, 53.1918) -> (-130.7121, 53.1918) projected
  line L12 (-130.7121, 53.1918) -> (-130.7121, 37.9418) projected
  arc A6 (-129.9621, 37.1918) -> (-130.7121, 37.9418) centre (-130.7121, 37.1918) ccw projected
  line L13 (-129.9621, 37.1918) -> (-125.4621, 37.1918) projected
  arc A7 (-124.7121, 36.4418) -> (-125.4621, 37.1918) centre (-124.7121, 37.1918) ccw projected
  line L14 (-124.7121, 36.4418) -> (-124.7121, 27.9418) projected
  arc A8 (-125.4621, 27.1918) -> (-124.7121, 27.9418) centre (-124.7121, 27.1918) ccw projected
  line L15 (-125.4621, 27.1918) -> (-129.9621, 27.1918) projected
  arc A9 (-130.7121, 26.4418) -> (-129.9621, 27.1918) centre (-130.7121, 27.1918) ccw projected
  line L16 (-130.7121, 26.4418) -> (-130.7121, 5.1918) projected
  line L17 (-130.7121, 5.1918) -> (-101.4621, 5.1918) projected
  arc A10 (-100.7121, 5.9418) -> (-101.4621, 5.1918) centre (-100.7121, 5.1918) ccw projected
  line L18 (-100.7121, 5.9418) -> (-100.7121, 10.4418) projected
  arc A11 (-99.9621, 11.1918) -> (-100.7121, 10.4418) centre (-100.7121, 11.1918) ccw projected
  line L19 (-99.9621, 11.1918) -> (-81.4621, 11.1918) projected
  circle A12 centre (-77.7121, 8.1918) radius 1.35 projected
  circle A13 centre (-103.7121, 8.1918) radius 1.35 projected
  circle A14 centre (-105.2121, 48.5918) radius 1.35 projected
  circle A15 centre (-83.2121, 48.5918) radius 1.35 projected
  circle A16 centre (-61.2121, 48.5918) radius 1.35 projected
  circle A17 centre (-55.9121, 42.2918) radius 1.35 projected
  circle A18 centre (-55.9121, 20.2918) radius 1.35 projected
  circle A19 centre (-61.2121, 13.9918) radius 1.35 projected
  circle A20 centre (-83.2121, 13.9918) radius 1.35 projected
  circle A21 centre (-105.2121, 13.9918) radius 1.35 projected
  line L20 (-118.5121, 16.5918) -> (-118.5121, 45.9918) projected
  line L21 (-118.5121, 45.9918) -> (-58.5121, 45.9918) projected
  line L22 (-58.5121, 45.9918) -> (-58.5121, 16.5918) projected
  line L23 (-58.5121, 16.5918) -> (-118.5121, 16.5918) projected
  circle A22 centre (-127.7121, 40.1918) radius 1.35 projected
  circle A23 centre (-127.7121, 24.1918) radius 1.35 projected
  circle A24 centre (-49.3121, 8.1918) radius 1.35 projected
  circle A25 centre (-23.3121, 8.1918) radius 1.35 projected
  line L24 (-7.6121, 38.9418) -> (-9.8121, 38.9418) projected
  line L25 (-9.8121, 38.9418) -> (-9.8121, 44.1418) projected
  line L26 (-9.8121, 44.1418) -> (-7.6121, 44.1418) projected
  line L27 (-7.6121, 44.1418) -> (-7.6121, 38.9418) projected
  line L28 (-7.6121, 14.5918) -> (-9.8121, 14.5918) projected
  line L29 (-9.8121, 14.5918) -> (-9.8121, 19.7918) projected
  line L30 (-9.8121, 19.7918) -> (-7.6121, 19.7918) projected
  line L31 (-7.6121, 19.7918) -> (-7.6121, 14.5918) projected
  line L32 (-95.7121, 5.1918) -> (-85.7121, 5.1918)
  line L33 (-85.7121, 5.1918) -> (-85.7121, 11.1918)
  line L34 (-85.7121, 11.1918) -> (-95.7121, 11.1918)
  line L35 (-95.7121, 11.1918) -> (-95.7121, 5.1918)
  line L36 (-95.7121, 5.1918) -> (-85.7121, 11.1918) construction
  line L37 (-85.7121, 5.1918) -> (-95.7121, 11.1918) construction
  line L38 (-41.3121, 5.1918) -> (-31.3121, 5.1918)
  line L39 (-31.3121, 5.1918) -> (-31.3121, 11.1918)
  line L40 (-31.3121, 11.1918) -> (-41.3121, 11.1918)
  line L41 (-41.3121, 11.1918) -> (-41.3121, 5.1918)
  line L42 (-41.3121, 5.1918) -> (-31.3121, 11.1918) construction
  line L43 (-31.3121, 5.1918) -> (-41.3121, 11.1918) construction
  line L44 (-130.7121, 53.1918) -> (-0.7121, 53.1918)
  line L45 (-0.7121, 53.1918) -> (-0.7121, 5.1918)
  line L46 (-0.7121, 5.1918) -> (-130.7121, 5.1918)
  line L47 (-130.7121, 5.1918) -> (-130.7121, 53.1918)
  point P0 (0, 0)
  point P1 (-90.7121, 8.1918)
  point P2 (-36.3121, 8.1918)
  dimension "d117" = 10
  dimension "d118" = 10
  constraints: 32 end point, 6 parallel, 4 midpoint, 3 horizontal, 3 perpendicular, 2 point on line
  measures "d117" distance of L34.end L33.end
  measures "d118" distance of L40.end L39.end
extrude "돌출14" add sketch "스케치15" against normal blind 6 contours L0 A1 L46 L33 L19 A0 | L35 L46 A10 L18 A11 L19 | A2 L2 A3 L3 L41 L46 | L39 L3 A4 L4 A5 L46
sketch "스케치17" plane through (6, 0, 0) normal (1, 0, 0) x (0, 0, -1)
  line L0 (-41.3121, 11.1918) -> (-31.3121, 11.1918) projected
  line L1 (-31.3121, 11.1918) -> (-31.3121, 5.1918) projected
  line L2 (-31.3121, 5.1918) -> (-0.7121, 5.1918) projected
  line L3 (-0.7121, 5.1918) -> (-0.7121, 24.1918) projected
  line L4 (-0.7121, 24.1918) -> (5.2879, 24.1918) projected
  line L5 (5.2879, 34.1918) -> (5.2879, 24.1918) projected
  line L6 (-0.7121, 34.1918) -> (5.2879, 34.1918) projected
  line L7 (-0.7121, 34.1918) -> (-0.7121, 53.1918) projected
  line L8 (-0.7121, 53.1918) -> (-130.7121, 53.1918) projected
  line L9 (-130.7121, 53.1918) -> (-130.7121, 37.9418) projected
  arc A0 (-129.9621, 37.1918) -> (-130.7121, 37.9418) centre (-130.7121, 37.1918) ccw projected
  line L10 (-129.9621, 37.1918) -> (-125.4621, 37.1918) projected
  arc A1 (-124.7121, 36.4418) -> (-125.4621, 37.1918) centre (-124.7121, 37.1918) ccw projected
  line L11 (-124.7121, 36.4418) -> (-124.7121, 27.9418) projected
  arc A2 (-125.4621, 27.1918) -> (-124.7121, 27.9418) centre (-124.7121, 27.1918) ccw projected
  line L12 (-125.4621, 27.1918) -> (-129.9621, 27.1918) projected
  arc A3 (-130.7121, 26.4418) -> (-129.9621, 27.1918) centre (-130.7121, 27.1918) ccw projected
  line L13 (-130.7121, 26.4418) -> (-130.7121, 5.1918) projected
  line L14 (-130.7121, 5.1918) -> (-95.7121, 5.1918) projected
  line L15 (-95.7121, 5.1918) -> (-95.7121, 11.1918) projected
  line L16 (-95.7121, 11.1918) -> (-85.7121, 11.1918) projected
  line L17 (-85.7121, 11.1918) -> (-85.7121, 5.1918) projected
  line L18 (-85.7121, 5.1918) -> (-41.3121, 5.1918) projected
  line L19 (-41.3121, 5.1918) -> (-41.3121, 11.1918) projected
  circle A4 centre (-77.7121, 8.1918) radius 1.35 projected
  circle A5 centre (-103.7121, 8.1918) radius 1.35 projected
  circle A6 centre (-105.2121, 48.5918) radius 1.35 projected
  circle A7 centre (-83.2121, 48.5918) radius 1.35 projected
  circle A8 centre (-61.2121, 48.5918) radius 1.35 projected
  circle A9 centre (-55.9121, 42.2918) radius 1.35 projected
  circle A10 centre (-55.9121, 20.2918) radius 1.35 projected
  circle A11 centre (-61.2121, 13.9918) radius 1.35 projected
  circle A12 centre (-83.2121, 13.9918) radius 1.35 projected
  circle A13 centre (-105.2121, 13.9918) radius 1.35 projected
  line L20 (-118.5121, 16.5918) -> (-118.5121, 45.9918) projected
  line L21 (-118.5121, 45.9918) -> (-58.5121, 45.9918) projected
  line L22 (-58.5121, 45.9918) -> (-58.5121, 16.5918) projected
  line L23 (-58.5121, 16.5918) -> (-118.5121, 16.5918) projected
  circle A14 centre (-127.7121, 40.1918) radius 1.35 projected
  circle A15 centre (-127.7121, 24.1918) radius 1.35 projected
  circle A16 centre (-49.3121, 8.1918) radius 1.35 projected
  circle A17 centre (-23.3121, 8.1918) radius 1.35 projected
  line L24 (-7.6121, 38.9418) -> (-9.8121, 38.9418) projected
  line L25 (-9.8121, 38.9418) -> (-9.8121, 44.1418) projected
  line L26 (-9.8121, 44.1418) -> (-7.6121, 44.1418) projected
  line L27 (-7.6121, 44.1418) -> (-7.6121, 38.9418) projected
  line L28 (-7.6121, 14.5918) -> (-9.8121, 14.5918) projected
  line L29 (-9.8121, 14.5918) -> (-9.8121, 19.7918) projected
  line L30 (-9.8121, 19.7918) -> (-7.6121, 19.7918) projected
  line L31 (-7.6121, 19.7918) -> (-7.6121, 14.5918) projected
  line L32 (-100.7121, 11.1918) -> (-80.7121, 11.1918)
  line L33 (-80.7121, 11.1918) -> (-80.7121, 5.1918)
  line L34 (-80.7121, 5.1918) -> (-100.7121, 5.1918)
  line L35 (-100.7121, 5.1918) -> (-100.7121, 11.1918)
  line L36 (-100.7121, 11.1918) -> (-80.7121, 5.1918) construction
  line L37 (-80.7121, 11.1918) -> (-100.7121, 5.1918) construction
  line L38 (-46.3121, 5.1918) -> (-26.3121, 5.1918)
  line L39 (-26.3121, 5.1918) -> (-26.3121, 11.1918)
  line L40 (-26.3121, 11.1918) -> (-46.3121, 11.1918)
  line L41 (-46.3121, 11.1918) -> (-46.3121, 5.1918)
  line L42 (-46.3121, 5.1918) -> (-26.3121, 11.1918) construction
  line L43 (-26.3121, 5.1918) -> (-46.3121, 11.1918) construction
  point P0 (0, 0)
  point P1 (-90.7121, 8.1918)
  point P2 (-36.3121, 8.1918)
  dimension "d132" = 20
  dimension "d133" = 20
  constraints: 24 end point, 4 midpoint, 4 parallel, 2 horizontal, 2 perpendicular, 2 point on line
  measures "d132" distance of L33.end L34.end
  measures "d133" distance of L40.end L39.end
extrude "돌출16" cut sketch "스케치17" against normal blind 10 contours L0 L1 L38 L19 | L19 L18 L41 L40 | L40 L39 L2 L1 | L18 L17 L32 L33 | L34 L15 L16 L17 | L14 L35 L32 L15
sketch "스케치18" plane through (6, 0, 0) normal (1, 0, 0) x (0, 0, -1)
  line L0 (-7.6121, 14.5918) -> (-9.8121, 14.5918) projected
  line L1 (-9.8121, 14.5918) -> (-9.8121, 19.7918) projected
  line L2 (-9.8121, 19.7918) -> (-7.6121, 19.7918) projected
  line L3 (-7.6121, 19.7918) -> (-7.6121, 14.5918) projected
  line L4 (-7.6121, 38.9418) -> (-9.8121, 38.9418) projected
  line L5 (-9.8121, 38.9418) -> (-9.8121, 44.1418) projected
  line L6 (-9.8121, 44.1418) -> (-7.6121, 44.1418) projected
  line L7 (-7.6121, 44.1418) -> (-7.6121, 38.9418) projected
  circle A0 centre (-23.3121, 8.1918) radius 1.35 projected
  circle A1 centre (-49.3121, 8.1918) radius 1.35 projected
  circle A2 centre (-127.7121, 24.1918) radius 1.35 projected
  circle A3 centre (-127.7121, 40.1918) radius 1.35 projected
  line L8 (-118.5121, 16.5918) -> (-118.5121, 45.9918) projected
  line L9 (-118.5121, 45.9918) -> (-58.5121, 45.9918) projected
  line L10 (-58.5121, 45.9918) -> (-58.5121, 16.5918) projected
  line L11 (-58.5121, 16.5918) -> (-118.5121, 16.5918) projected
  circle A4 centre (-105.2121, 13.9918) radius 1.35 projected
  circle A5 centre (-83.2121, 13.9918) radius 1.35 projected
  circle A6 centre (-61.2121, 13.9918) radius 1.35 projected
  circle A7 centre (-55.9121, 20.2918) radius 1.35 projected
  circle A8 centre (-55.9121, 42.2918) radius 1.35 projected
  circle A9 centre (-61.2121, 48.5918) radius 1.35 projected
  circle A10 centre (-83.2121, 48.5918) radius 1.35 projected
  circle A11 centre (-105.2121, 48.5918) radius 1.35 projected
  circle A12 centre (-103.7121, 8.1918) radius 1.35 projected
  circle A13 centre (-77.7121, 8.1918) radius 1.35 projected
  line L12 (-46.3121, 5.1918) -> (-46.3121, 11.1918) projected
  line L13 (-46.3121, 11.1918) -> (-26.3121, 11.1918) projected
  line L14 (-26.3121, 11.1918) -> (-26.3121, 5.1918) projected
  line L15 (-26.3121, 5.1918) -> (-0.7121, 5.1918) projected
  line L16 (-0.7121, 5.1918) -> (-0.7121, 24.1918) projected
  line L17 (-0.7121, 24.1918) -> (5.2879, 24.1918) projected
  line L18 (5.2879, 34.1918) -> (5.2879, 24.1918) projected
  line L19 (-0.7121, 34.1918) -> (5.2879, 34.1918) projected
  line L20 (-0.7121, 34.1918) -> (-0.7121, 53.1918) projected
  line L21 (-0.7121, 53.1918) -> (-130.7121, 53.1918) projected
  line L22 (-130.7121, 53.1918) -> (-130.7121, 37.9418) projected
  arc A14 (-129.9621, 37.1918) -> (-130.7121, 37.9418) centre (-130.7121, 37.1918) ccw projected
  line L23 (-129.9621, 37.1918) -> (-125.4621, 37.1918) projected
  arc A15 (-124.7121, 36.4418) -> (-125.4621, 37.1918) centre (-124.7121, 37.1918) ccw projected
  line L24 (-124.7121, 36.4418) -> (-124.7121, 27.9418) projected
  arc A16 (-125.4621, 27.1918) -> (-124.7121, 27.9418) centre (-124.7121, 27.1918) ccw projected
  line L25 (-125.4621, 27.1918) -> (-129.9621, 27.1918) projected
  arc A17 (-130.7121, 26.4418) -> (-129.9621, 27.1918) centre (-130.7121, 27.1918) ccw projected
  line L26 (-130.7121, 26.4418) -> (-130.7121, 5.1918) projected
  line L27 (-130.7121, 5.1918) -> (-100.7121, 5.1918) projected
  line L28 (-100.7121, 5.1918) -> (-100.7121, 11.1918) projected
  line L29 (-100.7121, 11.1918) -> (-80.7121, 11.1918) projected
  line L30 (-80.7121, 11.1918) -> (-80.7121, 5.1918) projected
  line L31 (-80.7121, 5.1918) -> (-46.3121, 5.1918) projected
  circle A18 centre (-100.7121, 11.1918) radius 0.75
  circle A19 centre (-80.7121, 11.1918) radius 0.75
  circle A20 centre (-46.3121, 11.1918) radius 0.75
  circle A21 centre (-26.3121, 11.1918) radius 0.75
  point P0 (0, 0)
  dimension "d136" = 1.5
  dimension "d137" = 1.5
  dimension "d138" = 1.5
  dimension "d139" = 1.5
  constraints: 4 centre point, 4 coincident
  measures "d136" diameter of A18
  measures "d137" diameter of A19
  measures "d138" diameter of A20
  measures "d139" diameter of A21
extrude "돌출17" cut sketch "스케치18" against normal blind 10 contours A20 L13 L12 | L12 L13 A20 | A19 L29 L30 | L30 L29 A19 | A21 L14 L13 | L13 L14 A21 | A18 L28 L29 | L29 L28 A18
